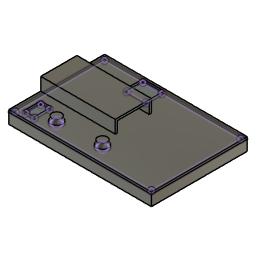
PCB housing v3 (Autodesk Fusion 360 design; units mm, degrees)
Autodesk Fusion 360 part; units mm, degrees
note: some values were not read from the file. Set by a fixed rule: which sketch regions a step uses.
sketch "Sketch1" plane through (0, 0, 0) normal (0, 0, 1) x (1, 0, 0)
  line L0 (0, 0) -> (64, 0)
  line L1 (64, 0) -> (64, 42)
  line L2 (64, 42) -> (0, 42)
  line L3 (0, 42) -> (0, 0)
  line L4 (18, 42) -> (27, 42)
  line L5 (27, 42) -> (27, 34.5)
  line L6 (27, 34.5) -> (18, 34.5)
  line L7 (18, 34.5) -> (18, 42)
  line L8 (3, 9) -> (7, 9)
  line L9 (7, 9) -> (7, 2)
  line L10 (7, 2) -> (3, 2)
  line L11 (3, 2) -> (3, 9)
  circle A0 centre (14.25, 5.25) radius 2.25
  circle A1 centre (34.75, 6.25) radius 2.25
  circle A2 centre (50, 33) radius 4.5
  line L12 (46.5, 15.5) -> (52.5, 15.5)
  line L13 (52.5, 15.5) -> (52.5, 11.5)
  line L14 (52.5, 11.5) -> (46.5, 11.5)
  line L15 (46.5, 11.5) -> (46.5, 15.5)
  line L16 (12, 7.5) -> (16.5, 7.5)
  line L17 (16.5, 7.5) -> (16.5, 3)
  line L18 (16.5, 3) -> (12, 3)
  line L19 (12, 3) -> (12, 7.5)
  line L20 (32.5, 8.5) -> (37, 8.5)
  line L21 (37, 8.5) -> (37, 4)
  line L22 (37, 4) -> (32.5, 4)
  line L23 (32.5, 4) -> (32.5, 8.5)
  dimension "d1" = 64
  dimension "d2" = 42
  dimension "d3" = 18
  dimension "d4" = 9
  dimension "d5" = 7.5
  dimension "d6" = 4
  dimension "d7" = 7
  dimension "d8" = 4.5
  dimension "d9" = 9
  dimension "d10" = 6
  dimension "d11" = 4
  dimension "d12" = 3
  dimension "d13" = 2
  dimension "d14" = 3
  dimension "d15" = 5
  dimension "d16" = 4
  dimension "d17" = 16
  dimension "d18" = 9
  dimension "d19" = 14
  dimension "d20" = 11.5
  dimension "d21" = 11.5
  constraint horizontal L0
  constraint vertical L1
  constraint horizontal L2
  constraint vertical L3
  constraint coincident L0.start L3.end
  constraint horizontal L4
  constraint vertical L5
  constraint horizontal L6
  constraint vertical L7
  constraint coincident L2 L4.start
  constraint horizontal L8
  constraint vertical L9
  constraint horizontal L10
  constraint vertical L11
  constraint horizontal L12
  constraint vertical L13
  constraint horizontal L14
  constraint vertical L15
  constraint equal A0 A1
  constraint horizontal L16
  constraint vertical L17
  constraint horizontal L18
  constraint vertical L19
  constraint tangent A0 L16
  constraint tangent A0 L19
  constraint tangent A0 L17
  constraint tangent A0 L18
  constraint horizontal L20
  constraint vertical L21
  constraint horizontal L22
  constraint vertical L23
  constraint tangent A1 L20
  constraint tangent A1 L21
  constraint tangent A1 L22
  constraint tangent A1 L23
  measures "d1" distance of L0.start L0.end
  measures "d2" distance of L0.start L2.end
  measures "d3" distance of L3 L7
  measures "d4" distance of L5.end L6.end
  measures "d5" distance of L4.end L5.end
  measures "d6" distance of L8.start L8.end
  measures "d7" distance of L8.start L10.end
  measures "d8" diameter of A0
  measures "d9" diameter of A2
  measures "d10" distance of L12.start L12.end
  measures "d11" distance of L12.end L13.end
  measures "d12" distance of L3 L11
  measures "d13" distance of L0 L10
  measures "d14" distance of L0 L18
  measures "d15" distance of L9 L19
  measures "d16" distance of L0 L22
  measures "d17" distance of L17 L23
  measures "d18" distance of L2 A2.centre
  measures "d19" distance of L1 A2.centre
  measures "d20" distance of L0 L14
  measures "d21" distance of L1 L13
extrude "Extrude1" add sketch "Sketch1" along normal blind 1 contours L0 L1 L2 L3 L5 L6 L7 | L2 L4 L5 L6 L7 | L8 L9 L10 L11 | A0 | A0 L17 L18 | A0 L16 L17 | A0 L16 L19 | A0 L18 L19 | A1 | A1 L21 L22 | A1 L20 L21 | A1 L20 L23 | A1 L22 L23 | A2 | L12 L13 L14 L15 makes body 1
extrude "Extrude2" add sketch "Sketch1" along normal blind 5 contours L2 L4 L5 L6 L7 bodies 1
extrude "Extrude3" add sketch "Sketch1" along normal blind 5 contours L8 L9 L10 L11 bodies 1
extrude "Extrude4" add sketch "Sketch1" along normal blind 3 contours A0 | A0 L17 L18 | A0 L16 L17 | A0 L16 L19 | A0 L18 L19 | A1 | A1 L21 L22 | A1 L20 L21 | A1 L20 L23 | A1 L22 L23 bodies 1
extrude "Extrude5" add sketch "Sketch1" along normal blind 5 from surface at 3 contours A0 | A1 bodies 1
extrude "Extrude6" add sketch "Sketch1" against normal blind 4 contours A2 bodies 1
extrude "Extrude7" add sketch "Sketch1" against normal blind 1.5 contours L12 L13 L14 L15 bodies 1
sketch "Sketch2" plane through (0, 0, 5) normal (0, 0, 1) x (-1, 0, 0)
  line L0 (-18, -34.5) -> (-27, -34.5)
  line L1 (-27, -34.5) -> (-27, -42)
  line L2 (-27, -42) -> (-18, -42)
  line L3 (-18, -42) -> (-18, -34.5)
  circle A0 centre (-34.75, -6.25) radius 2.25
  circle A1 centre (-14.25, -5.25) radius 2.25
  line L4 (-7, -9) -> (-3, -9)
  line L5 (-3, -9) -> (-3, -2)
  line L6 (-3, -2) -> (-7, -2)
  line L7 (-7, -2) -> (-7, -9)
  line L8 (-18, -42) -> (-18, -34.5)
  line L9 (-18, -34.5) -> (-27, -34.5)
  line L10 (-27, -34.5) -> (-27, -42)
  line L11 (-27, -42) -> (-18, -42)
  line L12 (-64, -42) -> (0, -42)
  line L13 (-64, 0) -> (-64, -42)
  line L14 (0, 0) -> (-64, 0)
  line L15 (0, -42) -> (0, 0)
  line L16 (0.5, 0.5) -> (-64.5, 0.5)
  line L17 (-64.5, 0.5) -> (-64.5, -42.5)
  line L18 (-64.5, -42.5) -> (0.5, -42.5)
  line L19 (0.5, -42.5) -> (0.5, 0.5)
  line L20 (1.5, 1.5) -> (-65.5, 1.5)
  line L21 (-65.5, 1.5) -> (-65.5, -43.5)
  line L22 (-65.5, -43.5) -> (1.5, -43.5)
  line L23 (1.5, -43.5) -> (1.5, 1.5)
  line L24 (-27.5, -42.5) -> (-17.5, -42.5)
  line L25 (-17.5, -42.5) -> (-17.5, -34)
  line L26 (-17.5, -34) -> (-27.5, -34)
  line L27 (-27.5, -34) -> (-27.5, -42.5)
  line L28 (-2.5, -1.5) -> (-7.5, -1.5)
  line L29 (-7.5, -1.5) -> (-7.5, -9.5)
  line L30 (-7.5, -9.5) -> (-2.5, -9.5)
  line L31 (-2.5, -9.5) -> (-2.5, -1.5)
  circle A2 centre (-14.25, -5.25) radius 2.75
  circle A3 centre (-34.75, -6.25) radius 2.75
  dimension "d37" = 0.5
  dimension "d38" = 1.5
  dimension "d39" = 0.5
  dimension "d42" = 0.5
  dimension "d43" = 0.5
  dimension "d44" = 0.5
extrude "Extrude8" add sketch "Sketch2" against normal up to surface (6 mm away) from surface at 1 separate body contours L20 L21 L22 L23 makes body 2
extrude "Extrude9" add sketch "Sketch2" against normal blind 1.5 from surface at 1 contours L12 L13 L14 L15 L25 L26 L27 | L12 L13 L14 L15 L16 L17 L18 L19 L25 L27 bodies 2
sketch "Sketch3" plane through (-1.5, 0, 0) normal (-1, 0, 0) x (0, -1, 0)
  line L0 (-43.5, 0) -> (1.5, 0)
  line L1 (1.5, 0) -> (1.5, 6)
  line L2 (1.5, 6) -> (-43.5, 6)
  line L3 (-43.5, 6) -> (-43.5, 0)
  line L4 (-9.5, 5) -> (-9.5, 1)
  line L5 (-9.5, 1) -> (-1.5, 1)
  line L6 (-1.5, 1) -> (-1.5, 5)
  line L7 (-9.5, 5) -> (-1.5, 5)
  point P0 (-9.5, 4.5)
  point P1 (-1.5, 4.5)
  point P2 (-2, 5)
  point P3 (-9, 5)
  dimension "d49" = 1
  constraint perpendicular L4 L5
  constraint vertical L6
  constraint coincident L4 P0
  measures "d49" distance of L0 L5
extrude "Extrude10" cut sketch "Sketch3" against normal up to surface (4 mm away) contours L4 L5 L6 L7 bodies 2
sketch "Sketch4" plane through (0, 43.5, 0) normal (0, 1, 0) x (-1, 0, 0)
  line L0 (-65.5, 0) -> (1.5, 0)
  line L1 (1.5, 0) -> (1.5, 6)
  line L2 (1.5, 6) -> (-65.5, 6)
  line L3 (-65.5, 6) -> (-65.5, 0)
  line L4 (-27.11, 5) -> (-17.5, 5)
  line L5 (-17.5, 5) -> (-17.5, 1)
  line L6 (-17.5, 1) -> (-27.11, 1)
  line L7 (-27.11, 1) -> (-27.11, 5)
  line L8 (-65.5, 5) -> (1.5, 5)
  point P0 (-17.5, 5)
  dimension "d52" = 1
  dimension "d55" = 1
  constraint horizontal L4
  constraint vertical L5
  constraint horizontal L6
  constraint vertical L7
  constraint coincident L7 L4.start
  constraint coincident L4.start L8
  constraint coincident L5 P0
  measures "d52" distance of L0 L6
  measures "d55" distance of L2 L4
extrude "Extrude11" cut sketch "Sketch4" against normal up to surface (1 mm away) contours L4 L5 L6 L7 L8 bodies 2
sketch "Sketch5" plane through (-1.5, 0, 0) normal (-1, 0, 0) x (0, -1, 0)
  line L0 (-9.5, 1) -> (-9.5, 5)
  line L1 (-9.5, 5) -> (-1.5, 5)
  line L2 (-1.5, 5) -> (-1.5, 1)
  line L3 (-1.5, 1) -> (-9.5, 1)
  line L4 (-43.5, 0) -> (1.5, 0)
  line L5 (1.5, 0) -> (1.5, 6)
  line L6 (1.5, 6) -> (-43.5, 6)
  line L7 (-43.5, 6) -> (-43.5, 0)
  line L8 (-30.5, 12) -> (-13.5, 12)
  line L9 (1.5, 6) -> (-30.5, 6)
  line L10 (-30.5, 6) -> (-30.5, 12)
  line L11 (-29.5, 11) -> (-14.5, 11)
  line L12 (-14.5, 11) -> (-14.5, 6)
  line L13 (-14.5, 6) -> (-29.5, 6)
  line L14 (-29.5, 6) -> (-29.5, 11)
  line L15 (-13.5, 12) -> (-13.5, 6)
  dimension "d56" = 15
  dimension "d59" = 1
  dimension "d60" = 5
  dimension "d61" = 1
  dimension "d62" = 1
  dimension "d63" = 15
  constraint horizontal L8
  constraint horizontal L9
  constraint vertical L10
  constraint coincident L5.end L6.start
  constraint horizontal L11
  constraint vertical L12
  constraint horizontal L13
  constraint vertical L14
  constraint coincident L9 L12.end
  constraint coincident L9 L15.end
  constraint vertical L15
  measures "d56" distance of L11.start L11.end
  measures "d59" distance of L12 L15
  measures "d60" distance of L11.start L13.end
  measures "d61" distance of L8 L11
  measures "d62" distance of L10 L14
  measures "d63" distance of L5 L15
extrude "Extrude12" add sketch "Sketch5" against normal blind 35 separate body contours L6 L8 L9 L10 L11 L12 L14 L15 makes body 3
